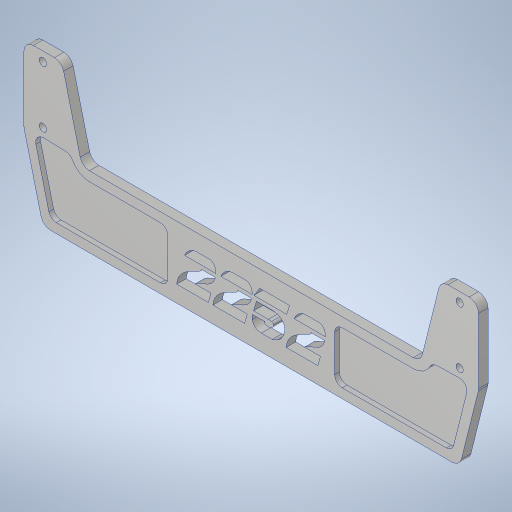
# Autodesk Inventor part: CL7-021
Saved by Autodesk Inventor 2023.4 (Build 274418000, 418)
## iProperties
Created: 2025-03-24
Part Number: CL7-021
Material: Aluminum 6061
Document SubType Name: Modeling
Designer: jmcintyr
Density: 2.7 g/cm^3
Appearance: Aluminum - Flat
Mass: 215.448 g
Surface Area: 424.682 cm^2
Volume: 79.7956 cm^3
Author: jmcintyr
Autodesk Inventor part; units mm, degrees
note: some values were not read from the file. Chosen so that the rebuilt part matches the saved one: direction of "Emboss1".
ref_plane "YZ Plane" through (0, 0, 0) normal (1, 0, 0) x (0, 1, 0)
ref_plane "XZ Plane" through (0, 0, 0) normal (0, 1, 0) x (-1, 0, 0)
ref_plane "XY Plane" through (0, 0, 0) normal (0, 0, 1) x (1, 0, 0)
sketch "Sketch1" plane through (0, 0, 0) normal (0, 0, 1) x (1, 0, 0)
  line L0 (152.4, 25.4) -> (-152.4, 25.4) construction
  line L1 (-152.4, 25.4) -> (-152.4, -25.4)
  line L2 (-152.4, -25.4) -> (152.4, -25.4) construction
  line L3 (152.4, -25.4) -> (152.4, 25.4)
  line L4 (152.4, 25.4) -> (-152.4, -25.4) construction
  line L5 (-152.4, 25.4) -> (152.4, -25.4) construction
  line L6 (-127, 25.4) -> (-127, -25.4) construction
  line L7 (127, 25.4) -> (127, -25.4) construction
  line L8 (-139.7, 19.05) -> (-139.7, -19.05) construction
  line L9 (139.7, 19.05) -> (139.7, -19.05) construction
  line L10 (-139.7, -76.2) -> (139.7, -76.2)
  line L11 (-152.4, -25.4) -> (-139.7, -76.2)
  line L12 (139.7, -76.2) -> (152.4, -25.4)
  line L13 (-127, 25.4) -> (-113.5062, -28.575)
  line L14 (127, 25.4) -> (113.5063, -28.575)
  line L15 (127, 25.4) -> (152.4, 25.4)
  line L16 (-152.4, 25.4) -> (-127, 25.4)
  line L17 (-113.5062, -28.575) -> (113.5063, -28.575)
  point P0 (0, 0)
  point P1 (-139.7, 0)
  point P2 (-152.4, 0)
  point P3 (0, -25.4)
  point P4 (0, -76.2)
  dimension "d0" = 304.8
  dimension "d1" = 50.8
  dimension "d2" = 25.4
  dimension "d3" = 25.4
  dimension "d4" = 38.1
  dimension "d5" = 12.7
  dimension "d6" = 12.7
  dimension "d8" = 279.4
  dimension "d18" = 47.625
  dimension "d19" = 3.175
  dimension "d21" = 101.6
  constraints: 36 end point, 6 midpoint, 4 coincident, 4 parallel, 4 point on line, 3 horizontal, 3 horizontal alignment, 3 perpendicular, 2 collinear, 2 vertical, 1 vertical alignment
  measures "d0" distance of L2.end L1.end
  measures "d1" distance of L1.end L0.end
  measures "d2" distance between parallel lines of L3 L7
  measures "d3" distance between parallel lines of L1 L6
  measures "d4" distance of L8.start L8.end
  measures "d5" distance between parallel lines of L6 L8
  measures "d6" distance between parallel lines of L3 L9
  measures "d8" distance of L10.start L10.end
  measures "d18" distance between parallel lines of L10 L17
  measures "d19" distance between parallel lines of L2 L17
  measures "d21" distance between parallel lines of L10 L0
extrude "Extrusion1" add sketch "Sketch1" against normal blind 6.35
hole "Hole1" at (-139.7, 19.05, 0) at (-139.7, -19.05, 0) at (139.7, -19.05, 0) at (139.7, 19.05, 0) direction (0, 0, -1) diameter 5.1054 end through all clearance for "Flat Head Machine Screw (82)" size "#10" standard "Ansi Unified Screw Threads"
fillet "Fillet1" radius 6.35 10 edges at (-113.5062, -28.575, -3.175) (-127, 25.4, -3.175) (-152.4, 25.4, -3.175) (-152.4, -25.4, -3.175) (-139.7, -76.2, -3.175) (139.7, -76.2, -3.175) (152.4, -25.4, -3.175) (152.4, 25.4, -3.175) (127, 25.4, -3.175) (113.5063, -28.575, -3.175)
sketch "Sketch2" plane through (0, 0, 0) normal (0, 0, 1) x (1, 0, 0)
  line L0 (-49.53, -39.6875) -> (49.53, -39.6875) construction
  line L1 (49.53, -39.6875) -> (49.53, -65.0875) construction
  line L2 (49.53, -65.0875) -> (-49.53, -65.0875) construction
  line L3 (-49.53, -65.0875) -> (-49.53, -39.6875) construction
  arc A0 (-114.7087, -23.7651) -> (-108.5483, -28.575) centre (-108.5483, -22.225) ccw construction
  line L4 (-108.5483, -28.575) -> (108.5483, -28.575) construction
  arc A1 (108.5483, -28.575) -> (114.7087, -23.7651) centre (108.5483, -22.225) ccw construction
  line L5 (114.7087, -23.7651) -> (125.7975, 20.5901) construction
  arc A2 (131.9579, 25.4) -> (125.7975, 20.5901) centre (131.9579, 19.05) ccw construction
  line L6 (131.9579, 25.4) -> (146.05, 25.4) construction
  arc A3 (152.4, 19.05) -> (146.05, 25.4) centre (146.05, 19.05) ccw construction
  line L7 (152.4, 19.05) -> (152.4, -24.6183) construction
  arc A4 (152.2104, -26.1584) -> (152.4, -24.6183) centre (146.05, -24.6183) ccw construction
  line L8 (152.2104, -26.1584) -> (140.9025, -71.3901) construction
  arc A5 (134.7421, -76.2) -> (140.9025, -71.3901) centre (134.7421, -69.85) ccw construction
  line L9 (134.7421, -76.2) -> (-134.7421, -76.2) construction
  arc A6 (-140.9025, -71.3901) -> (-134.7421, -76.2) centre (-134.7421, -69.85) ccw construction
  line L10 (-140.9025, -71.3901) -> (-152.2104, -26.1584) construction
  arc A7 (-152.4, -24.6183) -> (-152.2104, -26.1584) centre (-146.05, -24.6183) ccw construction
  line L11 (-152.4, -24.6183) -> (-152.4, 19.05) construction
  arc A8 (-146.05, 25.4) -> (-152.4, 19.05) centre (-146.05, 19.05) ccw construction
  line L12 (-146.05, 25.4) -> (-131.9579, 25.4) construction
  arc A9 (-125.7975, 20.5901) -> (-131.9579, 25.4) centre (-131.9579, 19.05) ccw construction
  line L13 (-125.7975, 20.5901) -> (-114.7087, -23.7651) construction
  circle A10 centre (139.7, -19.05) radius 2.5527 construction
  circle A11 centre (-139.7, 19.05) radius 2.5527 construction
  circle A12 centre (-139.7, -19.05) radius 2.5527 construction
  circle A13 centre (139.7, 19.05) radius 2.5527 construction
  line L14 (0, -28.575) -> (0, -76.2) construction
  line L15 (108.5483, -34.925) -> (-108.5483, -34.925)
  arc A14 (-120.8691, -25.3052) -> (-108.5483, -34.925) centre (-108.5483, -22.225) ccw
  line L16 (-120.8691, -25.3052) -> (-131.9579, 19.05) construction
  line L17 (-131.9579, 19.05) -> (-146.05, 19.05) construction
  line L18 (-146.05, 19.05) -> (-146.05, -24.6183) construction
  line L19 (-146.05, -24.6183) -> (-134.7421, -69.85)
  line L20 (-134.7421, -69.85) -> (134.7421, -69.85)
  line L21 (134.7421, -69.85) -> (146.05, -24.6183) construction
  line L22 (146.05, -24.6183) -> (146.05, 19.05) construction
  line L23 (146.05, 19.05) -> (131.9579, 19.05) construction
  line L24 (131.9579, 19.05) -> (120.8691, -25.3052) construction
  arc A15 (108.5483, -34.925) -> (120.8691, -25.3052) centre (108.5483, -22.225) ccw construction
  line L25 (-55.88, -33.3375) -> (55.88, -33.3375) construction
  line L26 (55.88, -33.3375) -> (55.88, -71.4375) construction
  line L27 (55.88, -71.4375) -> (-55.88, -71.4375) construction
  line L28 (-55.88, -71.4375) -> (-55.88, -33.3375)
  line L29 (-146.05, -24.6183) -> (-120.8691, -25.3052)
  line L30 (-49.9948, -65.1683) -> (-28.7574, -65.1279)
  line L31 (-28.7574, -65.1279) -> (-26.9792, -58.8638)
  line L32 (-26.9792, -58.8638) -> (-37.6686, -58.8638)
  spline S0 degree 2 poles (-37.6686, -58.8638) (-36.1329, -57.5706) (-28.7978, -54.7214) (-27.2823, -53.5898) knots 0 0 0 1 2 2 2
  spline S1 degree 2 poles (-27.2823, -53.5898) (-24.6554, -51.5287) (-23.9683, -48.2754) knots 0 0 0 1 1 1
  line L33 (-23.9683, -48.2754) -> (-33.2837, -48.2754)
  spline S2 degree 2 poles (-33.2837, -48.2754) (-33.2433, -48.3562) (-33.2433, -48.4573) knots 0 0 0 1 1 1
  spline S3 degree 2 poles (-33.2433, -48.4573) (-33.2433, -49.4878) (-37.0826, -51.3064) knots 0 0 0 1 1 1
  spline S4 degree 2 poles (-37.0826, -51.3064) (-42.7607, -53.9535) (-45.0845, -55.9136) knots 0 0 0 1 1 1
  spline S5 degree 2 poles (-45.0845, -55.9136) (-49.631, -59.6721) (-49.9948, -65.1683) knots 0 0 0 1 1 1
  spline S6 degree 2 poles (-23.6652, -45.8102) (-23.6652, -43.5268) (-24.3927, -42.2336) knots 0 0 0 1 1 1
  spline S7 degree 2 poles (-24.3927, -42.2336) (-25.8072, -39.6875) (-27.9087, -39.6875) knots 0 0 0 1 1 1
  line L34 (-27.9087, -39.6875) -> (-36.9411, -39.6875)
  spline S8 degree 2 poles (-36.9411, -39.6875) (-39.366, -39.6875) (-43.9125, -43.4056) (-44.7208, -45.8102) knots 0 0 0 1 2 2 2
  line L35 (-44.7208, -45.8102) -> (-23.6652, -45.8102)
  line L36 (-25.6859, -65.1683) -> (-4.4485, -65.1279)
  line L37 (-4.4485, -65.1279) -> (-2.6703, -58.8638)
  line L38 (-2.6703, -58.8638) -> (-13.3598, -58.8638)
  spline S9 degree 2 poles (-13.3598, -58.8638) (-11.824, -57.5706) (-4.489, -54.7214) (-2.9734, -53.5898) knots 0 0 0 1 2 2 2
  spline S10 degree 2 poles (-2.9734, -53.5898) (-0.3465, -51.5287) (0.3405, -48.2754) knots 0 0 0 1 1 1
  line L39 (0.3405, -48.2754) -> (-8.9749, -48.2754)
  spline S11 degree 2 poles (-8.9749, -48.2754) (-8.9345, -48.3562) (-8.9345, -48.4573) knots 0 0 0 1 1 1
  spline S12 degree 2 poles (-8.9345, -48.4573) (-8.9345, -49.4878) (-12.7738, -51.3064) knots 0 0 0 1 1 1
  spline S13 degree 2 poles (-12.7738, -51.3064) (-18.4519, -53.9535) (-20.7757, -55.9136) knots 0 0 0 1 1 1
  spline S14 degree 2 poles (-20.7757, -55.9136) (-25.3222, -59.6721) (-25.6859, -65.1683) knots 0 0 0 1 1 1
  spline S15 degree 2 poles (0.6436, -45.8102) (0.6436, -43.5268) (-0.0839, -42.2336) knots 0 0 0 1 1 1
  spline S16 degree 2 poles (-0.0839, -42.2336) (-1.4983, -39.6875) (-3.5998, -39.6875) knots 0 0 0 1 1 1
  line L40 (-3.5998, -39.6875) -> (-12.6323, -39.6875)
  spline S17 degree 2 poles (-12.6323, -39.6875) (-15.0571, -39.6875) (-19.6037, -43.4056) (-20.4119, -45.8102) knots 0 0 0 1 2 2 2
  line L41 (-20.4119, -45.8102) -> (0.6436, -45.8102)
  spline S18 degree 2 poles (11.4745, -54.8426) (13.0102, -54.8426) (13.6366, -54.9841) knots 0 0 0 1 1 1
  spline S19 degree 2 poles (13.6366, -54.9841) (14.9702, -55.3276) (14.9702, -56.3986) knots 0 0 0 1 1 1
  spline S20 degree 2 poles (14.9702, -56.3986) (14.9702, -57.4291) (13.4547, -59.0457) (12.3838, -59.1265) knots 0 0 0 1 2 2 2
  spline S21 degree 2 poles (12.3838, -59.1265) (11.6159, -59.1871) (11.1714, -59.1871) knots 0 0 0 1 1 1
  spline S22 degree 2 poles (11.1714, -59.1871) (9.0294, -59.1871) (9.0294, -57.8332) knots 0 0 0 1 1 1
  spline S23 degree 2 poles (9.0294, -57.8332) (9.0294, -57.5706) (9.0698, -57.3079) knots 0 0 0 1 1 1
  line L42 (9.0698, -57.3079) -> (0.8052, -57.3079)
  spline S24 degree 2 poles (0.8052, -57.3079) (0.4415, -59.6317) (0.6234, -60.4601) knots 0 0 0 1 1 1
  spline S25 degree 2 poles (0.6234, -60.4601) (1.5731, -65.1683) (6.8269, -65.1683) knots 0 0 0 1 1 1
  line L43 (6.8269, -65.1683) -> (14.0811, -65.1683)
  spline S26 degree 2 poles (14.0811, -65.1683) (15.7381, -64.9056) (17.6577, -63.6932) knots 0 0 0 1 1 1
  spline S27 degree 2 poles (17.6577, -63.6932) (19.3551, -62.6223) (20.123, -61.6321) knots 0 0 0 1 1 1
  spline S28 degree 2 poles (20.123, -61.6321) (22.0426, -59.1467) (22.4468, -55.9742) knots 0 0 0 1 1 1
  spline S29 degree 2 poles (22.4468, -55.9742) (22.4872, -55.5499) (22.4872, -55.1457) knots 0 0 0 1 1 1
  spline S30 degree 2 poles (22.4872, -55.1457) (22.4872, -52.923) (21.3152, -51.4883) knots 0 0 0 1 1 1
  spline S31 degree 2 poles (21.3152, -51.4883) (19.9007, -49.6495) (16.1826, -48.2754) (13.4951, -48.2754) knots 0 0 0 1 2 2 2
  line L44 (13.4951, -48.2754) -> (3.4725, -48.2754)
  line L45 (3.4725, -48.2754) -> (1.5731, -54.8426)
  line L46 (1.5731, -54.8426) -> (11.4745, -54.8426)
  line L47 (23.7804, -45.8102) -> (1.7752, -45.8102)
  line L48 (1.7752, -45.8102) -> (5.6751, -39.6875)
  line L49 (5.6751, -39.6875) -> (25.6192, -39.6875)
  line L50 (25.6192, -39.6875) -> (23.7804, -45.8102)
  line L51 (23.4167, -65.1683) -> (44.6541, -65.1279)
  line L52 (44.6541, -65.1279) -> (46.4323, -58.8638)
  line L53 (46.4323, -58.8638) -> (35.7429, -58.8638)
  spline S32 degree 2 poles (35.7429, -58.8638) (37.2786, -57.5706) (44.6137, -54.7214) (46.1292, -53.5898) knots 0 0 0 1 2 2 2
  spline S33 degree 2 poles (46.1292, -53.5898) (48.7561, -51.5287) (49.4431, -48.2754) knots 0 0 0 1 1 1
  line L54 (49.4431, -48.2754) -> (40.1278, -48.2754)
  spline S34 degree 2 poles (40.1278, -48.2754) (40.1682, -48.3562) (40.1682, -48.4573) knots 0 0 0 1 1 1
  spline S35 degree 2 poles (40.1682, -48.4573) (40.1682, -49.4878) (36.3289, -51.3064) knots 0 0 0 1 1 1
  spline S36 degree 2 poles (36.3289, -51.3064) (30.6507, -53.9535) (28.327, -55.9136) knots 0 0 0 1 1 1
  spline S37 degree 2 poles (28.327, -55.9136) (23.7804, -59.6721) (23.4167, -65.1683) knots 0 0 0 1 1 1
  spline S38 degree 2 poles (49.7462, -45.8102) (49.7462, -43.5268) (49.0188, -42.2336) knots 0 0 0 1 1 1
  spline S39 degree 2 poles (49.0188, -42.2336) (47.6043, -39.6875) (45.5028, -39.6875) knots 0 0 0 1 1 1
  line L55 (45.5028, -39.6875) -> (36.4703, -39.6875)
  spline S40 degree 2 poles (36.4703, -39.6875) (34.0455, -39.6875) (29.499, -43.4056) (28.6907, -45.8102) knots 0 0 0 1 2 2 2
  line L56 (28.6907, -45.8102) -> (49.7462, -45.8102)
  point P0 (0, 0)
  point P1 (0, -39.6875)
  point P2 (-49.53, -52.3875)
  point P3 (0, -52.3875)
  point P4 (-55.88, -69.85)
  point P5 (-55.88, -34.925)
  dimension "d22" = 25.4
  dimension "d23" = 99.06
  dimension "d26" = 6.35
  dimension "d27" = 6.35
  constraints: 32 end point, 5 midpoint, 4 point on circle, 2 centre point, 1 horizontal, 1 horizontal alignment, 1 vertical alignment, 16 other
  measures "d22" distance of L2.end L0.start
  measures "d23" distance of L1.end L2.end
  measures "d26" distance between parallel lines of L4 L15
  measures "d27" distance between parallel lines of L3 L28
extrude "Extrusion2" cut sketch "Sketch2" against normal blind 3.175 contours L28 L20 L19 L29 A14 L15
emboss "Emboss1" sketch "Sketch2" operation cut depth 6.35 direction (0, 0, -1) contours S5 S4 S3 S2 L33 S1 S0 L32 L31 L30 | L35 S8 L34 S7 S6 | S14 S13 S12 S11 L39 S10 S9 L38 L37 L36 | L41 S17 L40 S16 S15 | L46 L45 L44 S31 S30 S29 S28 S27 S26 L43 S25 S24 L42 S23 S22 S21 S20 S19 S18 | L47 L48 L49 L50 | S37 S36 S35 S34 L54 S33 S32 L53 L52 L51 | L56 S40 L55 S39 S38
fillet "Fillet2" radius 5.08 5 edges at (-146.05, -24.6183, -1.5875) (-120.8691, -25.3052, -1.5875) (-55.88, -34.925, -1.5875) (-55.88, -69.85, -1.5875) (-134.7421, -69.85, -1.5875)
mirror "Mirror1" about plane through (0, 0, 0) normal (1, 0, 0) of "Extrusion2", "Fillet2"
equation "\"d3\" = d2"
equation "\"d6\" = d5"
equation "\"d27\" = d26"
body "Solid1"
